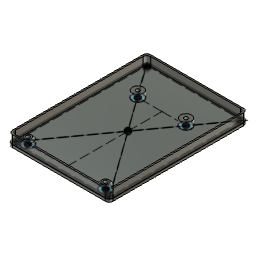
WCH CH32V307V Bumper Case (Autodesk Fusion 360 design; units mm, degrees)
Autodesk Fusion 360 part; units mm, degrees
sketch "Sketch1" plane through (0, 0, 0) normal (0, 0, 1) x (1, 0, 0)
  line L0 (37.06, -51.77) -> (-37.06, -51.77) construction
  line L1 (-37.06, -51.77) -> (-37.06, 51.77) construction
  line L2 (-37.06, 51.77) -> (37.06, 51.77) construction
  line L3 (37.06, 51.77) -> (37.06, -51.77) construction
  line L4 (37.06, -51.77) -> (-37.06, 51.77) construction
  line L5 (-37.06, -51.77) -> (37.06, 51.77) construction
  line L6 (36.26, 53.97) -> (-36.26, 53.97)
  line L7 (-39.26, 50.97) -> (-39.26, -50.97)
  line L8 (-36.26, -53.97) -> (36.26, -53.97)
  line L9 (39.26, -50.97) -> (39.26, 50.97)
  line L10 (39.26, 53.97) -> (-39.26, -53.97) construction
  line L11 (-39.26, 53.97) -> (39.26, -53.97) construction
  arc A0 (-36.26, 53.97) -> (-39.26, 50.97) centre (-36.26, 50.97) ccw
  arc A1 (39.26, 50.97) -> (36.26, 53.97) centre (36.26, 50.97) ccw
  arc A2 (-39.26, -50.97) -> (-36.26, -53.97) centre (-36.26, -50.97) ccw
  arc A3 (36.26, -53.97) -> (39.26, -50.97) centre (36.26, -50.97) ccw
  line L12 (35.06, -52.77) -> (-35.06, -52.77)
  line L13 (-38.06, -49.77) -> (-38.06, 49.77)
  line L14 (-35.06, 52.77) -> (35.06, 52.77)
  line L15 (38.06, 49.77) -> (38.06, -49.77)
  line L16 (38.06, -52.77) -> (-38.06, 52.77) construction
  line L17 (-38.06, -52.77) -> (38.06, 52.77) construction
  arc A4 (-35.06, 52.77) -> (-38.06, 49.77) centre (-35.06, 49.77) ccw
  arc A5 (38.06, 49.77) -> (35.06, 52.77) centre (35.06, 49.77) ccw
  arc A6 (35.06, -52.77) -> (38.06, -49.77) centre (35.06, -49.77) ccw
  arc A7 (-38.06, -49.77) -> (-35.06, -52.77) centre (-35.06, -49.77) ccw
  line L18 (0, 0) -> (0, 26.51) construction
  line L19 (0, 26.51) -> (-18.83, 26.51) construction
  line L20 (0, 26.51) -> (18.83, 26.51) construction
  line L21 (0, 0) -> (0, -47.9) construction
  line L22 (0, -47.9) -> (-30.4, -47.9) construction
  line L23 (0, -47.9) -> (30.4, -47.9) construction
  circle A8 centre (-18.83, 26.51) radius 1.51
  circle A9 centre (18.83, 26.51) radius 1.51
  circle A10 centre (-18.83, 26.51) radius 4.25
  circle A11 centre (18.83, 26.51) radius 4.25
  line L24 (-16.03, 28.1266) -> (-18.83, 29.7432)
  line L25 (-18.83, 29.7432) -> (-21.63, 28.1266)
  line L26 (-21.63, 28.1266) -> (-21.63, 24.8934)
  line L27 (-21.63, 24.8934) -> (-18.83, 23.2768)
  line L28 (-18.83, 23.2768) -> (-16.03, 24.8934)
  line L29 (-16.03, 24.8934) -> (-16.03, 28.1266)
  line L30 (16.03, 24.8934) -> (18.83, 23.2768)
  line L31 (18.83, 23.2768) -> (21.63, 24.8934)
  line L32 (21.63, 24.8934) -> (21.63, 28.1266)
  line L33 (21.63, 28.1266) -> (18.83, 29.7432)
  line L34 (18.83, 29.7432) -> (16.03, 28.1266)
  line L35 (16.03, 28.1266) -> (16.03, 24.8934)
  circle A12 centre (-30.4, -47.9) radius 1.51
  circle A13 centre (-30.4, -47.9) radius 4.25
  line L36 (-27.6, -46.2834) -> (-30.4, -44.6668)
  line L37 (-30.4, -44.6668) -> (-33.2, -46.2834)
  line L38 (-33.2, -46.2834) -> (-33.2, -49.5166)
  line L39 (-33.2, -49.5166) -> (-30.4, -51.1332)
  line L40 (-30.4, -51.1332) -> (-27.6, -49.5166)
  line L41 (-27.6, -49.5166) -> (-27.6, -46.2834)
  circle A14 centre (30.4, -47.9) radius 1.51
  circle A15 centre (30.4, -47.9) radius 4.25
  line L42 (27.6, -49.5166) -> (30.4, -51.1332)
  line L43 (30.4, -51.1332) -> (33.2, -49.5166)
  line L44 (33.2, -49.5166) -> (33.2, -46.2834)
  line L45 (33.2, -46.2834) -> (30.4, -44.6668)
  line L46 (30.4, -44.6668) -> (27.6, -46.2834)
  line L47 (27.6, -46.2834) -> (27.6, -49.5166)
  point P0 (-18.83, 26.51)
  point P1 (18.83, 26.51)
  point P2 (-30.4, -47.9)
  point P3 (30.4, -47.9)
  dimension "d21" = 74.12
  dimension "d22" = 103.54
  dimension "d23" = 78.52
  dimension "d24" = 107.94
  dimension "d25" = 3
  dimension "d26" = 3
  dimension "d27" = 3
  dimension "d28" = 3
  dimension "d29" = 76.12
  dimension "d30" = 105.54
  dimension "d31" = 3
  dimension "d32" = 3
  dimension "d33" = 3
  dimension "d34" = 3
  dimension "d35" = 26.51
  dimension "d36" = 18.83
  dimension "d37" = 18.83
  dimension "d38" = 47.9
  dimension "d39" = 30.4
  dimension "d40" = 30.4
  dimension "d41" = 3.02
  dimension "d42" = 3.02
  dimension "d43" = 8.5
  dimension "d44" = 8.5
  dimension "d45" = 2.8
  dimension "d46" = 2.8
  dimension "d47" = 3.02
  dimension "d48" = 8.5
  dimension "d49" = 2.8
  dimension "d50" = 3.02
  dimension "d51" = 8.5
  dimension "d52" = 2.8
  constraint horizontal L0
  constraint perpendicular L0 L1
  constraint parallel L0 L2
  constraint parallel L1 L3
  constraint coincident L4 L18.start
  constraint coincident L5 L18.start
  constraint coincident L18.start L21.start
  constraint horizontal L6
  constraint perpendicular L6 L7
  constraint parallel L6 L8
  constraint parallel L7 L9
  constraint coincident L10 L18.start
  constraint coincident L11 L18.start
  constraint coincident L11.start L7
  constraint coincident L11.start L6
  constraint tangent L7 A0
  constraint tangent L6 A0
  constraint coincident L10.start L6
  constraint coincident L10.start L9
  constraint tangent L6 A1
  constraint tangent L9 A1
  constraint coincident L10.end L7
  constraint coincident L10.end L8
  constraint tangent L7 A2
  constraint tangent L8 A2
  constraint coincident L11.end L8
  constraint coincident L11.end L9
  constraint tangent L8 A3
  constraint tangent L9 A3
  constraint horizontal L12
  constraint perpendicular L12 L13
  constraint parallel L12 L14
  constraint parallel L13 L15
  constraint coincident L16 L18.start
  constraint coincident L17 L18.start
  constraint coincident L16.end L13
  constraint coincident L16.end L14
  constraint tangent L13 A4
  constraint tangent L14 A4
  constraint coincident L17.end L14
  constraint coincident L17.end L15
  constraint tangent L14 A5
  constraint tangent L15 A5
  constraint coincident L16.start L12
  constraint coincident L16.start L15
  constraint tangent L12 A6
  constraint tangent L15 A6
  constraint coincident L17.start L12
  constraint coincident L17.start L13
  constraint tangent L12 A7
  constraint tangent L13 A7
  constraint vertical L18
  constraint perpendicular L18 L19
  constraint perpendicular L18 L20
  constraint vertical L21
  constraint perpendicular L21 L22
  constraint perpendicular L21 L23
  constraint coincident P0 L19.end
  constraint coincident P1 L20.end
  constraint concentric A8 A10
  constraint concentric A9 A11
  constraint coincident P2 L22.end
  constraint concentric A12 A13
  constraint coincident P3 L23.end
  constraint concentric A14 A15
  measures "d21" distance of L1.end L2.end
  measures "d22" distance of L0.end L1.end
  measures "d23" distance of L10.end L11.end
  measures "d24" distance of L11.start L10.end
  measures "d25" radius of A0
  measures "d26" radius of A1
  measures "d27" radius of A2
  measures "d28" radius of A3
  measures "d29" distance of L16.end L17.end
  measures "d30" distance of L17.start L16.end
  measures "d31" radius of A4
  measures "d32" radius of A5
  measures "d33" radius of A6
  measures "d34" radius of A7
  measures "d35" distance of L18.start L18.end
  measures "d36" distance of L18.end P0
  measures "d37" distance of L18.end P1
  measures "d38" distance of L18.start L21.end
  measures "d39" distance of L21.end P2
  measures "d40" distance of L21.end P3
  measures "d41" diameter of A8
  measures "d42" diameter of A9
  measures "d43" diameter of A10
  measures "d44" diameter of A11
  measures "d45" distance of P0 L29
  measures "d46" distance of P1 L35
  measures "d47" diameter of A12
  measures "d48" diameter of A13
  measures "d49" distance of P2 L41
  measures "d50" diameter of A14
  measures "d51" diameter of A15
  measures "d52" distance of P3 L47
extrude "Extrude1" add sketch "Sketch1" against normal blind 2.26 contours L6 L7 L8 L9 A0 A1 A2 A3 | L12 L13 L14 L15 A4 A5 A6 A7 | A10 | A11 | A13 | A15
extrude "Extrude2" add sketch "Sketch1" along normal blind 6.6 contours L6 L7 L8 L9 A0 A1 A2 A3
extrude "Extrude3" add sketch "Sketch1" along normal blind 5 contours A10 | A11 | L24 L25 L26 L27 L28 L29 | L30 L31 L32 L33 L34 L35 | A13 | L36 L37 L38 L39 L40 L41 | A15 | L42 L43 L44 L45 L46 L47
chamfer "Chamfer1" distance 0.61 angle 45 4 edges at (28.9922, -47.354, 0) (17.4222, 27.056, 0) (-20.2378, 27.056, 0) (-31.8078, -47.354, 0)
chamfer "Chamfer2" distance 1.61 angle 45 2 edges at (-34.3624, -49.4369, 5) (26.4376, -49.4369, 5)
equation "BoardLength = 103.54 mm"
equation "BoardWidth = 74.12 mm"
equation "BoardFillet = 3 mm"
equation "CaseOffset = 1 mm"
equation "NutSize = ( 5.6 / 2 ) * 1 mm"
equation "NutDepth = 2.26 mm"
equation "HoleDiameter = 3.02 mm"
equation "UpperHolesLength = 26.51 mm"
equation "UpperHolesWidth = 37.66 mm"
equation "LowerHolesLength = 47.9 mm"
equation "LowerHolesWidth = 60.8 mm"
equation "StandoffDiameter = 8.5 mm"
equation "StandoffHeight = 5 mm"
equation "PCBHeight = 1.6 mm"
equation "CaseWallWidth = 1.2 mm"
equation "CaseLength = BoardLength + ( CaseOffset * 2 ) + ( CaseWallWidth * 2 )"
equation "CaseWidth = BoardWidth + ( CaseOffset * 2 ) + ( CaseWallWidth * 2 )"
equation "BumperLength = BoardLength + ( CaseOffset * 2 )"
equation "BumperWidth = BoardWidth + ( CaseOffset * 2 )"
equation "BoltChamfer = floor(( NutSize / ( sqrt(3) / 2 ) / 2 ) * 100) / 100"
equation "d21 = BoardWidth"
equation "d22 = BoardLength"
equation "d23 = CaseWidth"
equation "d24 = CaseLength"
equation "d25 = BoardFillet"
equation "d26 = BoardFillet"
equation "d27 = BoardFillet"
equation "d28 = BoardFillet"
equation "d29 = BumperWidth"
equation "d30 = BumperLength"
equation "d31 = BoardFillet"
equation "d32 = BoardFillet"
equation "d33 = BoardFillet"
equation "d34 = BoardFillet"
equation "d35 = UpperHolesLength"
equation "d36 = UpperHolesWidth / 2"
equation "d37 = UpperHolesWidth / 2"
equation "d38 = LowerHolesLength"
equation "d39 = LowerHolesWidth / 2"
equation "d40 = LowerHolesWidth / 2"
equation "d41 = HoleDiameter"
equation "d42 = HoleDiameter"
equation "d43 = StandoffDiameter"
equation "d44 = StandoffDiameter"
equation "d45 = NutSize"
equation "d46 = NutSize"
equation "d47 = HoleDiameter"
equation "d48 = StandoffDiameter"
equation "d49 = NutSize"
equation "d50 = HoleDiameter"
equation "d51 = StandoffDiameter"
equation "d52 = NutSize"
equation "d53 = -NutDepth"
equation "d55 = StandoffHeight + PCBHeight"
equation "d57 = StandoffHeight"
equation "d59 = BoltChamfer - 1 mm"
equation "d60 = BoltChamfer"
